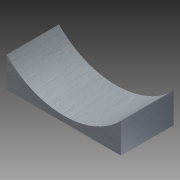
# Autodesk Inventor part: Thurst_Duct_Support
Saved by Autodesk Inventor 2011 SP1 (Build 150282100, 282)
## iProperties
Created: 2011-06-11
Part Number: Thurst_Duct_Support
Document SubType Name: Modeling
Designer: Andrew G. Meyer
Mass: 190.666 g
Surface Area: 335.727 cm^2
Volume: 190.666 cm^3
Density: 1 g/cm^3
Author: Andrew G. Meyer
Autodesk Inventor part; units mm, degrees
ref_plane "YZ Plane" through (0, 0, 0) normal (1, 0, 0) x (0, 1, 0)
ref_plane "XZ Plane" through (0, 0, 0) normal (0, 1, 0) x (-1, 0, 0)
ref_plane "XY Plane" through (0, 0, 0) normal (0, 0, 1) x (1, 0, 0)
sketch "Sketch1" plane through (0, 0, 0) normal (0, 0, 1) x (1, 0, 0)
  line L0 (-34.979, 58.0913) -> (-34.979, 17.9974)
  line L1 (-34.979, 17.9974) -> (117.421, 17.9974)
  line L2 (117.421, 17.9974) -> (117.421, 58.0913)
  arc A0 (-34.979, 58.0913) -> (117.421, 58.0913) centre (41.221, 132.2974) ccw
  point P0 (0, 0)
  dimension "d0" = 106.3625
  dimension "d1" = 152.4
  dimension "d2" = 7.9375
  constraints: 6 end point, 2 perpendicular, 2 point on circle, 1 centre point, 1 parallel, 1 vertical
  measures "d0" radius of A0
  measures "d1" distance of L0.end L1.end
  measures "d2" distance edge to line of A0 L1
extrude "Extrusion1" add sketch "Sketch1" along normal blind 69.85
body "Solid1"
